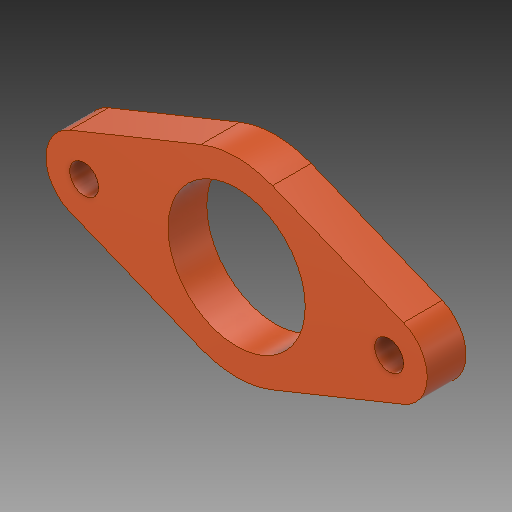
# Autodesk Inventor part: IRClamp
Saved by Autodesk Inventor 2017 (Build 210142000, 142)
## iProperties
Created: 2017-02-15
Part Number: IRClamp
Material: Phenolic Resin
Document SubType Name: Modeling
Designer: Moonlight.Admin
Density: 1.38 g/cm^3
Appearance: Smooth - Light Orange
Author: Moonlight.Admin
Autodesk Inventor part; units mm, degrees
ref_plane "YZ Plane" through (0, 0, 0) normal (1, 0, 0) x (0, 1, 0)
ref_plane "XZ Plane" through (0, 0, 0) normal (0, 1, 0) x (-1, 0, 0)
ref_plane "XY Plane" through (0, 0, 0) normal (0, 0, 1) x (1, 0, 0)
derived "CombinedHousingV2.ipt"
sketch "IR Distance" plane through (0, 0, 0) normal (0, 0, 1) x (1, 0, 0)
  line L0 (36.2, -29.125) -> (36.2, -50.625) construction
  line L1 (56.625, -24.13) -> (30.125, -24.13) construction
  circle A0 centre (12.7, 42) radius 9
  circle A1 centre (12.7, 42) radius 12.5
  circle A2 centre (-7.3, 42) radius 5
  circle A3 centre (32.7, 42) radius 5
  circle A4 centre (-7.3, 42) radius 1.905
  circle A5 centre (32.7, 42) radius 1.905
  circle A6 centre (-7.3, 42) radius 3.4925
  circle A7 centre (32.7, 42) radius 3.4925
  point P0 (0, 0)
sketch "Sketch2" plane through (0, 0, 0) normal (0, 0, 1) x (1, 0, 0)
  circle A0 centre (-7.3, 42) radius 5 construction
  circle A1 centre (12.7, 42) radius 12.5 construction
  circle A2 centre (32.7, 42) radius 5 construction
  circle A3 centre (12.7, 42) radius 9 projected
  line L0 (-9.175, 46.6351) -> (8.0125, 53.5878)
  line L1 (17.3875, 53.5878) -> (34.575, 46.6351)
  line L2 (34.575, 37.3649) -> (17.3875, 30.4122)
  line L3 (8.0125, 30.4122) -> (-9.175, 37.3649)
  arc A4 (-9.175, 46.6351) -> (-9.175, 37.3649) centre (-7.3, 42) ccw
  arc A5 (34.575, 37.3649) -> (34.575, 46.6351) centre (32.7, 42) ccw
  arc A6 (17.3875, 53.5878) -> (8.0125, 53.5878) centre (12.7, 42) ccw
  arc A7 (8.0125, 30.4122) -> (17.3875, 30.4122) centre (12.7, 42) ccw
  circle A8 centre (-7.3, 42) radius 1.905 projected
  circle A9 centre (32.7, 42) radius 1.905 projected
  point P0 (0, 0)
  constraints: 16 point on circle, 8 end point, 8 tangent, 5 concentric, 4 centre point
extrude "Extrusion1" add sketch "Sketch2" along normal blind 5.08
body "Solid1"
